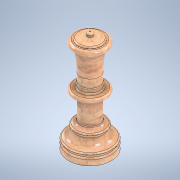
# Autodesk Inventor part: królowa
Saved by Autodesk Inventor 2021 (Build 250183000, 183)
## iProperties
Created: 2021-01-07
Part Number: królowa
Material: Drewno (brzoza)
Document SubType Name: Modeling
Designer: Adam
Density: 0.55 g/cm^3
Appearance: Brzoza — naturalna — polerowana
Author: Adam
Autodesk Inventor part; units mm, degrees
ref_plane "YZ Plane" through (0, 0, 0) normal (1, 0, 0) x (0, 1, 0)
ref_plane "XZ Plane" through (0, 0, 0) normal (0, 1, 0) x (-1, 0, 0)
ref_plane "XY Plane" through (0, 0, 0) normal (0, 0, 1) x (1, 0, 0)
sketch "Szkic1" plane through (0, 0, 0) normal (1, 0, 0) x (0, 1, 0)
  line L0 (2, 8) -> (2, -8)
  line L1 (2, 8) -> (78, 8)
  line L2 (2, -8) -> (7, -8)
  line L3 (7, -8) -> (7, -7)
  line L4 (7, -7) -> (8, -7)
  line L5 (8, -7) -> (8, -8)
  line L6 (8, -8) -> (10, -8)
  arc A0 (16, -2) -> (10, -8) centre (16, -8) ccw
  line L7 (16, -2) -> (17, -2)
  line L8 (17, -2) -> (17, -3)
  line L9 (17, -3) -> (19, -3)
  arc A1 (21, 1) -> (19, -3) centre (24, -3) ccw
  line L10 (21, 1) -> (39, 1)
  line L11 (39, 1) -> (39, -4)
  line L12 (39, -4) -> (42, -4)
  line L13 (42, -4) -> (42, 0)
  line L14 (42, 0) -> (43, 0)
  line L15 (43, 0) -> (43, 1)
  line L16 (43, 1) -> (45, 1)
  line L17 (45, 1) -> (45, 0.5)
  line L18 (45, 0.5) -> (46, 0.5)
  line L19 (46, 0.5) -> (46, 1)
  line L20 (46, 1) -> (49, 1)
  line L21 (49, 1) -> (52, 1)
  line L22 (74, -1) -> (75, 7)
  line L23 (74, -1) -> (73, -1)
  line L24 (73, -1) -> (73, -4)
  line L25 (73, -4) -> (69, -4)
  line L26 (69, -4) -> (69, -1)
  arc A2 (69, -1) -> (52, 1) centre (52, -72.25) ccw
  line L27 (75, 7) -> (74.875, 6)
  line L28 (75, 7) -> (75, 6)
  line L29 (75, 6) -> (78, 6)
  line L30 (78, 6) -> (78, 8)
  point P0 (0, 0)
  constraints: 62 end point, 13 perpendicular, 6 point on circle, 5 horizontal, 5 point on line, 4 vertical, 3 centre point, 1 tangent
revolve "Obrót2" add sketch "Szkic1" angle 360 about axis through (0, 2, 8) along (0, 1, 0)
fillet "Zaokrąglenie1" radius 1 1 edges at (0, 7, 24)
fillet "Zaokrąglenie2" radius 1 2 edges at (0, 8, 24) (0, 10, 24)
fillet "Zaokrąglenie3" radius 1 2 edges at (0, 17, 19) (0, 19, 19)
fillet "Zaokrąglenie4" radius 1 1 edges at (0, 21, 15)
fillet "Zaokrąglenie5" radius 1.5 2 edges at (0, 39, 20) (0, 42, 20)
fillet "Zaokrąglenie6" radius 1 1 edges at (0, 43, 16)
fillet "Zaokrąglenie7" radius 0.5 2 edges at (0, 45, 15.5) (0, 46, 15.5)
fillet "Zaokrąglenie8" radius 2 2 edges at (0, 69, 20) (0, 73, 20)
fillet "Zaokrąglenie9" radius 1 1 edges at (0, 74, 17)
fillet "Zaokrąglenie10" radius 1.5 1 edges at (0, 78, 10)
fillet "Zaokrąglenie11" radius 0.5 1 edges at (0, 75, 10)
